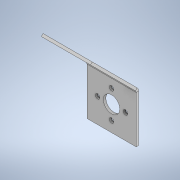
# Autodesk Inventor part: head
Saved by Autodesk Inventor 2022 (Build 260153000, 153)
## iProperties
Created: 2022-10-18
Part Number: head
Material: 一般
Document SubType Name: Sheet Metal
Designer: haya
Density: 1 g/cm^3
Sheet Metal Rule: Default_mm
Appearance: 既定
Author: haya
Autodesk Inventor part; units mm, degrees
ref_plane "YZ Plane" through (0, 0, 0) normal (1, 0, 0) x (0, 1, 0)
ref_plane "XZ Plane" through (0, 0, 0) normal (0, 1, 0) x (-1, 0, 0)
ref_plane "XY Plane" through (0, 0, 0) normal (0, 0, 1) x (1, 0, 0)
sketch "スケッチ2" plane through (0, 0, 0) normal (0, 0, 1) x (1, 0, 0)
  line L0 (0, 0) -> (30, 0)
  line L1 (30, 0) -> (30, 30)
  line L2 (30, 30) -> (0, 30)
  line L3 (0, 30) -> (0, 0)
  dimension "d0" = 30
  dimension "d1" = 30
  measures "d0" distance of L0.start L0.end
  measures "d1" distance of L2.end L0.start
extrude "プレート1" add sketch "スケッチ2" along normal blind 1.5
sketch "スケッチ5" plane through (0, 28.9393, 1.0607) normal (0, 0.7071068, -0.7071068) x (-1, 0, 0)
  line L0 (-30, 0) -> (0, 0)
  line L1 (0, 0) -> (0, 40)
  line L2 (0, 40) -> (-30, 40)
  line L3 (-30, 40) -> (-30, 0)
  constraints: 6 end point, 1 horizontal, 1 perpendicular, 1 vertical
edge flange "フランジ1" height 40 angle 45 thickness 1.5 bend radius 1.5 thickness toward (0, 0.7071068, -0.7071068) relief tear relief width 1.5 relief depth 0.75 edges at (15, 30, 1.5) wall of the first edge with corners at (30, 28.9393, 1.0607) (0, 28.9393, 1.0607) (0, 57.2236, 29.3449) (30, 57.2236, 29.3449)
bend "曲げ1"
corner "コーナー1"
sketch "スケッチ6" plane through (0, 0, 1.5) normal (0, 0, 1) x (1, 0, 0)
  line L0 (30, 0) -> (0, 0) projected
  line L1 (15, 0) -> (15, 28.7574) construction
  line L2 (30, 28.7574) -> (0, 28.7574) projected
  line L3 (0, 0) -> (0, 28.7574) projected
  line L4 (0, 15) -> (30, 15) construction
  point P0 (15, 15)
  dimension "d34" = 15
  constraints: 4 end point, 3 midpoint, 1 horizontal, 1 point on line
  measures "d34" distance between parallel lines of L4 L0
hole "穴3" at (15, 15, 1.5) direction (0, 0, -1) diameter 10 end through all
sketch "スケッチ7" plane through (0, 0, 1.5) normal (0, 0, 1) x (1, 0, 0)
  circle A0 centre (15, 15) radius 5 projected
  line L0 (30, 28.7574) -> (0, 28.7574) projected
  line L1 (0, 0) -> (0, 28.7574) projected
  line L2 (30, 0) -> (0, 0) projected
  line L3 (30, 28.7574) -> (30, 0) projected
  line L4 (15, 15) -> (30, 15) construction
  line L5 (30, 0) -> (30, 28.7574) projected
  line L6 (15, 15) -> (15, 30) construction
  line L7 (15, 15) -> (0, 15) construction
  line L8 (15, 15) -> (15, 0) construction
  point P0 (23.5, 15)
  point P1 (15, 23.5)
  point P2 (6.5, 15)
  point P3 (15, 6.5)
  dimension "d42" = 8.5
  dimension "d45" = 360
  constraints: 8 end point, 5 point on line, 2 coincident, 1 horizontal, 15 other
  measures "d42" distance of point (23.5, 15) L4.start
hole "穴4" at (23.5, 15, 1.5) at (15, 23.5, 1.5) at (6.5, 15, 1.5) at (15, 6.5, 1.5) direction (0, 0, -1) diameter 2.8 end through all
sketch "スケッチ8" plane through (0, 57.2236, 29.3449) normal (0, -0.7071068, 0.7071068) x (1, 0, 0)
  line L0 (30, 0) -> (0, 0) projected
  line L1 (15, 0) -> (15, -38.7574) construction
  line L2 (0, -38.7574) -> (30, -38.7574) projected
  line L3 (0, -38.7574) -> (0, 0) projected
  line L4 (0, -15) -> (29.8306, -15) construction
  point P0 (0, -61.2132)
  point P1 (14.9153, -15)
  dimension "d54" = 15
  constraints: 4 end point, 3 midpoint, 1 horizontal, 1 point on line
  measures "d54" distance between parallel lines of L4 L0
hole "穴5" at (14.9153, 46.617, 18.7383) direction (0, 0.7071068, -0.7071068) diameter 20 end through all
equation "\"d23\" = Thickness"
equation "\"d24\" = BendReliefWidth"
equation "\"d25\" = BendReliefDepth"
equation "\"d26\" = MinimumRemnant"
equation "\"d27\" = TransitionRadius"
equation "\"d30\" = BendRadius"
equation "\"d31\" = CornerReliefSize"
equation "\"d32\" = GapSize"
equation "\"d33\" = JacobiRadiusSize"
equation "\"BendRadius\" = Thickness"
equation "\"BendReliefWidth\" = Thickness"
equation "\"BendReliefDepth\" = 0.5 * Thickness"
equation "\"CornerReliefSize\" = 4 * Thickness"
equation "\"MinimumRemnant\" = 2 * Thickness"
equation "\"TransitionRadius\" = BendRadius"
equation "\"JacobiRadiusSize\" = BendRadius"
equation "\"GapSize\" = Thickness"
equation "\"Thickness\" = 1.5"
